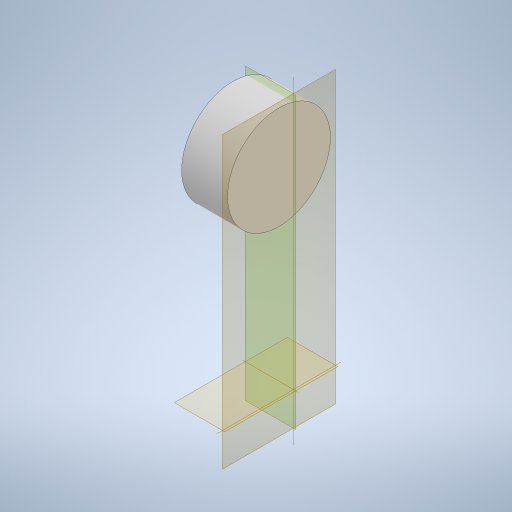
# Autodesk Inventor part: HTW-000166
Saved by Autodesk Inventor 2024.4 (Build 284460000, 460)
## iProperties
Created: 2025-11-13
Part Number: HTW-000166
Material: Generisch
Document SubType Name: Modeling
Designer: s0598146
Density: 1 g/cm^3
Appearance: Vorgabe
Author: s0598146
Autodesk Inventor part; units mm, degrees
sketch "Skizze1" plane through (0, 0, 0) normal (1, 0, 0) x (0, 1, 0)
  circle A0 centre (-0.628, 8.6983) radius 2.2366
  line L0 (-0.628, 9.8147) -> (-2.256, 9.1635)
  line L1 (-2.256, 9.1635) -> (-1.442, 8.3727)
  line L2 (-1.442, 8.3727) -> (-0.628, 9.8147)
  line L3 (0.7173, 9.2142) -> (-0.628, 6.8313)
  line L4 (-0.628, 6.8313) -> (0.127, 9.3885)
  line L5 (0.127, 9.3885) -> (0.7173, 9.2142)
  point P0 (0, 0)
  constraints: 12 end point, 1 centre point, 1 parallel, 1 perpendicular
extrude "Extrusion1" add sketch "Skizze1" against normal blind 2 contours A0 | L2 L1 L0 | L3 L4 L5
